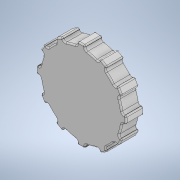
# Autodesk Inventor part: Dial_Radio
Saved by Autodesk Inventor 2021 (Build 250183000, 183)
## iProperties
Created: 2021-05-07
Part Number: Dial_Radio
Material: Generic
Document SubType Name: Modeling
Designer: trent
Density: 1 g/cm^3
Appearance: Default
Author: trent
Autodesk Inventor part; units mm, degrees
ref_plane "YZ Plane" through (0, 0, 0) normal (1, 0, 0) x (0, 1, 0)
ref_plane "XZ Plane" through (0, 0, 0) normal (0, 1, 0) x (-1, 0, 0)
ref_plane "XY Plane" through (0, 0, 0) normal (0, 0, 1) x (1, 0, 0)
sketch "Sketch1" plane through (0, 0, 0) normal (0, 0, 1) x (1, 0, 0)
  arc A0 (0.4789, 8.7369) -> (-0.5192, 8.7346) centre (0, 0) ccw
  line L0 (0.7133, 8.4304) -> (0.715, 8.4785)
  line L1 (-0.7524, 8.4247) -> (-0.7542, 8.4763)
  arc A1 (-0.5192, 8.7346) -> (-0.7542, 8.4763) centre (-0.5044, 8.485) ccw
  arc A2 (0.715, 8.4785) -> (0.4789, 8.7369) centre (0.4652, 8.4873) ccw
  arc A3 (-1.1785, 7.9127) -> (-0.7524, 8.4247) centre (-1.2521, 8.4073) ccw
  arc A4 (0.7133, 8.4304) -> (1.1417, 7.9181) centre (1.213, 8.413) ccw
  line L2 (-3.5975, 7.6577) -> (-3.62, 7.7001)
  line L3 (-4.864, 6.9198) -> (-4.8913, 6.9636)
  arc A5 (-4.8169, 7.3048) -> (-4.8913, 6.9636) centre (-4.6793, 7.0961) ccw
  arc A6 (-3.62, 7.7001) -> (-3.9537, 7.8058) centre (-3.8408, 7.5828) ccw
  arc A7 (-4.9769, 6.2634) -> (-4.864, 6.9198) centre (-5.288, 6.6549) ccw
  arc A8 (-3.9537, 7.8058) -> (-4.8169, 7.3048) centre (0, 0) ccw
  arc A9 (-3.5975, 7.6577) -> (-2.9703, 7.4281) centre (-3.156, 7.8924) ccw
  line L4 (-6.9443, 4.833) -> (-6.9851, 4.8585)
  line L5 (-7.6722, 3.5607) -> (-7.7178, 3.585)
  arc A10 (-7.824, 3.9176) -> (-7.7178, 3.585) centre (-7.6004, 3.8057) ccw
  arc A11 (-6.9851, 4.8585) -> (-7.3269, 4.7831) centre (-7.1176, 4.6465) ccw
  arc A12 (-7.4419, 2.9358) -> (-7.6722, 3.5607) centre (-7.907, 3.1193) ccw
  arc A13 (-7.3269, 4.7831) -> (-7.824, 3.9176) centre (0, 0) ccw
  arc A14 (-6.9443, 4.833) -> (-6.2864, 4.9478) centre (-6.6794, 5.257) ccw
  line L6 (-8.4304, 0.7133) -> (-8.4785, 0.715)
  line L7 (-8.4247, -0.7524) -> (-8.4763, -0.7542)
  arc A15 (-8.7346, -0.5192) -> (-8.4763, -0.7542) centre (-8.485, -0.5044) ccw
  arc A16 (-8.4785, 0.715) -> (-8.7369, 0.4789) centre (-8.4873, 0.4652) ccw
  arc A17 (-7.9127, -1.1785) -> (-8.4247, -0.7524) centre (-8.4073, -1.2521) ccw
  arc A18 (-8.7369, 0.4789) -> (-8.7346, -0.5192) centre (0, 0) ccw
  arc A19 (-8.4304, 0.7133) -> (-7.9181, 1.1417) centre (-8.413, 1.213) ccw
  line L8 (-7.6577, -3.5975) -> (-7.7001, -3.62)
  line L9 (-6.9198, -4.864) -> (-6.9636, -4.8913)
  arc A20 (-7.3048, -4.8169) -> (-6.9636, -4.8913) centre (-7.0961, -4.6793) ccw
  arc A21 (-7.7001, -3.62) -> (-7.8058, -3.9537) centre (-7.5828, -3.8408) ccw
  arc A22 (-6.2634, -4.9769) -> (-6.9198, -4.864) centre (-6.6549, -5.288) ccw
  arc A23 (-7.8058, -3.9537) -> (-7.3048, -4.8169) centre (0, 0) ccw
  arc A24 (-7.6577, -3.5975) -> (-7.4281, -2.9703) centre (-7.8924, -3.156) ccw
  line L10 (-4.833, -6.9443) -> (-4.8585, -6.9851)
  line L11 (-3.5607, -7.6722) -> (-3.585, -7.7178)
  arc A25 (-3.9176, -7.824) -> (-3.585, -7.7178) centre (-3.8057, -7.6004) ccw
  arc A26 (-4.8585, -6.9851) -> (-4.7831, -7.3269) centre (-4.6465, -7.1176) ccw
  arc A27 (-2.9358, -7.4419) -> (-3.5607, -7.6722) centre (-3.1193, -7.907) ccw
  arc A28 (-4.7831, -7.3269) -> (-3.9176, -7.824) centre (0, 0) ccw
  arc A29 (-4.833, -6.9443) -> (-4.9478, -6.2864) centre (-5.257, -6.6794) ccw
  line L12 (-0.7133, -8.4304) -> (-0.715, -8.4785)
  line L13 (0.7524, -8.4247) -> (0.7542, -8.4763)
  arc A30 (0.5192, -8.7346) -> (0.7542, -8.4763) centre (0.5044, -8.485) ccw
  arc A31 (-0.715, -8.4785) -> (-0.4789, -8.7369) centre (-0.4652, -8.4873) ccw
  arc A32 (1.1785, -7.9127) -> (0.7524, -8.4247) centre (1.2521, -8.4073) ccw
  arc A33 (-0.4789, -8.7369) -> (0.5192, -8.7346) centre (0, 0) ccw
  arc A34 (-0.7133, -8.4304) -> (-1.1417, -7.9181) centre (-1.213, -8.413) ccw
  line L14 (3.5975, -7.6577) -> (3.62, -7.7001)
  line L15 (4.864, -6.9198) -> (4.8913, -6.9636)
  arc A35 (4.8169, -7.3048) -> (4.8913, -6.9636) centre (4.6793, -7.0961) ccw
  arc A36 (3.62, -7.7001) -> (3.9537, -7.8058) centre (3.8408, -7.5828) ccw
  arc A37 (4.9769, -6.2634) -> (4.864, -6.9198) centre (5.288, -6.6549) ccw
  arc A38 (3.9537, -7.8058) -> (4.8169, -7.3048) centre (0, 0) ccw
  arc A39 (3.5975, -7.6577) -> (2.9703, -7.4281) centre (3.156, -7.8924) ccw
  line L16 (6.9443, -4.833) -> (6.9851, -4.8585)
  line L17 (7.6722, -3.5607) -> (7.7178, -3.585)
  arc A40 (7.824, -3.9176) -> (7.7178, -3.585) centre (7.6004, -3.8057) ccw
  arc A41 (6.9851, -4.8585) -> (7.3269, -4.7831) centre (7.1176, -4.6465) ccw
  arc A42 (7.4419, -2.9358) -> (7.6722, -3.5607) centre (7.907, -3.1193) ccw
  arc A43 (7.3269, -4.7831) -> (7.824, -3.9176) centre (0, 0) ccw
  arc A44 (6.9443, -4.833) -> (6.2864, -4.9478) centre (6.6794, -5.257) ccw
  line L18 (8.4304, -0.7133) -> (8.4785, -0.715)
  line L19 (8.4247, 0.7524) -> (8.4763, 0.7542)
  arc A45 (8.7346, 0.5192) -> (8.4763, 0.7542) centre (8.485, 0.5044) ccw
  arc A46 (8.4785, -0.715) -> (8.7369, -0.4789) centre (8.4873, -0.4652) ccw
  arc A47 (7.9127, 1.1785) -> (8.4247, 0.7524) centre (8.4073, 1.2521) ccw
  arc A48 (8.7369, -0.4789) -> (8.7346, 0.5192) centre (0, 0) ccw
  arc A49 (8.4304, -0.7133) -> (7.9181, -1.1417) centre (8.413, -1.213) ccw
  line L20 (7.6577, 3.5975) -> (7.7001, 3.62)
  line L21 (6.9198, 4.864) -> (6.9636, 4.8913)
  arc A50 (7.3048, 4.8169) -> (6.9636, 4.8913) centre (7.0961, 4.6793) ccw
  arc A51 (7.7001, 3.62) -> (7.8058, 3.9537) centre (7.5828, 3.8408) ccw
  arc A52 (6.2634, 4.9769) -> (6.9198, 4.864) centre (6.6549, 5.288) ccw
  arc A53 (7.8058, 3.9537) -> (7.3048, 4.8169) centre (0, 0) ccw
  arc A54 (7.6577, 3.5975) -> (7.4281, 2.9703) centre (7.8924, 3.156) ccw
  line L22 (4.833, 6.9443) -> (4.8585, 6.9851)
  line L23 (3.5607, 7.6722) -> (3.585, 7.7178)
  arc A55 (3.9176, 7.824) -> (3.585, 7.7178) centre (3.8057, 7.6004) ccw
  arc A56 (4.8585, 6.9851) -> (4.7831, 7.3269) centre (4.6465, 7.1176) ccw
  arc A57 (2.9358, 7.4419) -> (3.5607, 7.6722) centre (3.1193, 7.907) ccw
  arc A58 (4.7831, 7.3269) -> (3.9176, 7.824) centre (0, 0) ccw
  arc A59 (4.833, 6.9443) -> (4.9478, 6.2864) centre (5.257, 6.6794) ccw
  arc A60 (-1.1785, 7.9127) -> (-2.9703, 7.4281) centre (0, 0) ccw
  arc A61 (-4.9769, 6.2634) -> (-6.2864, 4.9478) centre (0, 0) ccw
  arc A62 (-7.4419, 2.9358) -> (-7.9181, 1.1417) centre (0, 0) ccw
  arc A63 (-7.9127, -1.1785) -> (-7.4281, -2.9703) centre (0, 0) ccw
  arc A64 (-6.2634, -4.9769) -> (-4.9478, -6.2864) centre (0, 0) ccw
  arc A65 (-2.9358, -7.4419) -> (-1.1417, -7.9181) centre (0, 0) ccw
  arc A66 (1.1785, -7.9127) -> (2.9703, -7.4281) centre (0, 0) ccw
  arc A67 (4.9769, -6.2634) -> (6.2864, -4.9478) centre (0, 0) ccw
  arc A68 (7.4419, -2.9358) -> (7.9181, -1.1417) centre (0, 0) ccw
  arc A69 (7.9127, 1.1785) -> (7.4281, 2.9703) centre (0, 0) ccw
  arc A70 (6.2634, 4.9769) -> (4.9478, 6.2864) centre (0, 0) ccw
  arc A71 (2.9358, 7.4419) -> (1.1417, 7.9181) centre (0, 0) ccw
  point P0 (0.7235, 8.72)
  point P1 (-0.7626, 8.7167)
  point P2 (0.6972, 7.9696)
  point P3 (-0.7364, 7.966)
  point P4 (-3.7335, 7.9135)
  point P5 (-5.0188, 7.1676)
  point P6 (-7.1901, 4.9865)
  point P7 (-7.9302, 3.6979)
  point P8 (-8.72, 0.7235)
  point P9 (-8.7167, -0.7626)
  point P10 (-7.9135, -3.7335)
  point P11 (-7.1676, -5.0188)
  point P12 (-4.9865, -7.1901)
  point P13 (-3.6979, -7.9302)
  point P14 (-0.7235, -8.72)
  point P15 (0.7626, -8.7167)
  point P16 (3.7335, -7.9135)
  point P17 (5.0188, -7.1676)
  point P18 (7.1901, -4.9865)
  point P19 (7.9302, -3.6979)
  point P20 (8.72, -0.7235)
  point P21 (8.7167, 0.7626)
  point P22 (7.9135, 3.7335)
  point P23 (7.1676, 5.0188)
  point P24 (4.9865, 7.1901)
  point P25 (3.6979, 7.9302)
  dimension "d1" = 17.5
  dimension "d4" = 0.25
  dimension "d5" = 0.5
  dimension "d8" = 360
  dimension "d10" = 8
  dimension "d11" = 4
  dimension "d12" = 0.8374
  dimension "d13" = 0.9159
  dimension "d14" = 8.4077
  dimension "d15" = 8.3542
  constraints: 168 point on circle, 72 centre point, 48 end point, 26 point on line, 8 tangent, 2 coincident, 2 equal radius, 265 other
  measures "d1" diameter of A0
  measures "d4" radius of A1
  measures "d5" radius of A3
  measures "d10" radius of A71
  measures "d11" angle of L18 L19
  measures "d12" distance between parallel lines of L18 L6
  measures "d13" distance between parallel lines of L7 L19
  measures "d14" distance from line of point (0.697, 7.97) L18
  measures "d15" distance from line of point (-0.736, 7.966) L18
extrude "Extrusion1" add sketch "Sketch1" along normal blind 3.5
fillet "Fillet1" radius 0.25 96 edges at (7.1493, 4.9236, 3.5) (6.9417, 4.8776, 3.5) (6.5701, 4.7952, 3.5) (5.6437, 5.67, 3.5) (4.7645, 6.5934, 3.5) (4.8457, 6.9647, 3.5) (4.8906, 7.1714, 3.5) (4.3575, 7.5878, 3.5) (3.7297, 7.8386, 3.5) (3.5729, 7.695, 3.5) (3.2922, 7.4378, 3.5) (2.0526, 7.7322, 3.5) (0.8294, 8.0923, 3.5) (0.7142, 8.4545, 3.5) (0.6497, 8.6559, 3.5) (-0.0202, 8.75, 3.5) (-0.6893, 8.6533, 3.5) (-0.7533, 8.4505, 3.5) (-0.8678, 8.0875, 3.5) (-2.0885, 7.7226, 3.5) (-3.3278, 7.4228, 3.5) (-3.6087, 7.6789, 3.5) (-3.7653, 7.8211, 3.5) (-4.3925, 7.5676, 3.5) (-4.9236, 7.1493, 3.5) (-4.8776, 6.9417, 3.5) (-4.7952, 6.5701, 3.5) (-5.67, 5.6437, 3.5) (-6.5934, 4.7645, 3.5) (-6.9647, 4.8457, 3.5) (-7.1714, 4.8906, 3.5) (-7.5878, 4.3575, 3.5) (-7.8386, 3.7297, 3.5) (-7.695, 3.5729, 3.5) (-7.4378, 3.2922, 3.5) (-7.7322, 2.0526, 3.5) (-8.0923, 0.8294, 3.5) (-8.4545, 0.7142, 3.5) (-8.6559, 0.6497, 3.5) (-8.75, -0.0202, 3.5) (-8.6533, -0.6893, 3.5) (-8.4505, -0.7533, 3.5) (-8.0875, -0.8678, 3.5) (-7.7226, -2.0885, 3.5) (-7.4228, -3.3278, 3.5) (-7.6789, -3.6087, 3.5) (-7.8211, -3.7653, 3.5) (-7.5676, -4.3925, 3.5) (-7.1493, -4.9236, 3.5) (-6.9417, -4.8776, 3.5) (-6.5701, -4.7952, 3.5) (-5.6437, -5.67, 3.5) (-4.7645, -6.5934, 3.5) (-4.8457, -6.9647, 3.5) (-4.8906, -7.1714, 3.5) (-4.3575, -7.5878, 3.5) (-3.7297, -7.8386, 3.5) (-3.5729, -7.695, 3.5) (-3.2922, -7.4378, 3.5) (-2.0526, -7.7322, 3.5) (-0.8294, -8.0923, 3.5) (-0.7142, -8.4545, 3.5) (-0.6497, -8.6559, 3.5) (0.0202, -8.75, 3.5) (0.6893, -8.6533, 3.5) (0.7533, -8.4505, 3.5) (0.8678, -8.0875, 3.5) (2.0885, -7.7226, 3.5) (3.3278, -7.4228, 3.5) (3.6087, -7.6789, 3.5) (3.7653, -7.8211, 3.5) (4.3925, -7.5676, 3.5) (4.9236, -7.1493, 3.5) (4.8776, -6.9417, 3.5) (4.7952, -6.5701, 3.5) (5.67, -5.6437, 3.5) (6.5934, -4.7645, 3.5) (6.9647, -4.8457, 3.5) (7.1714, -4.8906, 3.5) (7.5878, -4.3575, 3.5) (7.8386, -3.7297, 3.5) (7.695, -3.5729, 3.5) (7.4378, -3.2922, 3.5) (7.7322, -2.0526, 3.5) (8.0923, -0.8294, 3.5) (8.4545, -0.7142, 3.5) (8.6559, -0.6497, 3.5) (8.75, 0.0202, 3.5) (8.6533, 0.6893, 3.5) (8.4505, 0.7533, 3.5) (8.0875, 0.8678, 3.5) (7.7226, 2.0885, 3.5) (7.4228, 3.3278, 3.5) (7.6789, 3.6087, 3.5) (7.8211, 3.7653, 3.5) (7.5676, 4.3925, 3.5)
fillet "Fillet2" radius 0.25 96 edges at (7.1493, 4.9236, 0) (6.9417, 4.8776, 0) (6.5701, 4.7952, 0) (5.6437, 5.67, 0) (4.7645, 6.5934, 0) (4.8457, 6.9647, 0) (4.8906, 7.1714, 0) (4.3575, 7.5878, 0) (3.7297, 7.8386, 0) (3.5729, 7.695, 0) (3.2922, 7.4378, 0) (2.0526, 7.7322, 0) (0.8294, 8.0923, 0) (0.7142, 8.4545, 0) (0.6497, 8.6559, 0) (-0.0202, 8.75, 0) (-0.6893, 8.6533, 0) (-0.7533, 8.4505, 0) (-0.8678, 8.0875, 0) (-2.0885, 7.7226, 0) (-3.3278, 7.4228, 0) (-3.6087, 7.6789, 0) (-3.7653, 7.8211, 0) (-4.3925, 7.5676, 0) (-4.9236, 7.1493, 0) (-4.8776, 6.9417, 0) (-4.7952, 6.5701, 0) (-5.67, 5.6437, 0) (-6.5934, 4.7645, 0) (-6.9647, 4.8457, 0) (-7.1714, 4.8906, 0) (-7.5878, 4.3575, 0) (-7.8386, 3.7297, 0) (-7.695, 3.5729, 0) (-7.4378, 3.2922, 0) (-7.7322, 2.0526, 0) (-8.0923, 0.8294, 0) (-8.4545, 0.7142, 0) (-8.6559, 0.6497, 0) (-8.75, -0.0202, 0) (-8.6533, -0.6893, 0) (-8.4505, -0.7533, 0) (-8.0875, -0.8678, 0) (-7.7226, -2.0885, 0) (-7.4228, -3.3278, 0) (-7.6789, -3.6087, 0) (-7.8211, -3.7653, 0) (-7.5676, -4.3925, 0) (-7.1493, -4.9236, 0) (-6.9417, -4.8776, 0) (-6.5701, -4.7952, 0) (-5.6437, -5.67, 0) (-4.7645, -6.5934, 0) (-4.8457, -6.9647, 0) (-4.8906, -7.1714, 0) (-4.3575, -7.5878, 0) (-3.7297, -7.8386, 0) (-3.5729, -7.695, 0) (-3.2922, -7.4378, 0) (-2.0526, -7.7322, 0) (-0.8294, -8.0923, 0) (-0.7142, -8.4545, 0) (-0.6497, -8.6559, 0) (0.0202, -8.75, 0) (0.6893, -8.6533, 0) (0.7533, -8.4505, 0) (0.8678, -8.0875, 0) (2.0885, -7.7226, 0) (3.3278, -7.4228, 0) (3.6087, -7.6789, 0) (3.7653, -7.8211, 0) (4.3925, -7.5676, 0) (4.9236, -7.1493, 0) (4.8776, -6.9417, 0) (4.7952, -6.5701, 0) (5.67, -5.6437, 0) (6.5934, -4.7645, 0) (6.9647, -4.8457, 0) (7.1714, -4.8906, 0) (7.5878, -4.3575, 0) (7.8386, -3.7297, 0) (7.695, -3.5729, 0) (7.4378, -3.2922, 0) (7.7322, -2.0526, 0) (8.0923, -0.8294, 0) (8.4545, -0.7142, 0) (8.6559, -0.6497, 0) (8.75, 0.0202, 0) (8.6533, 0.6893, 0) (8.4505, 0.7533, 0) (8.0875, 0.8678, 0) (7.7226, 2.0885, 0) (7.4228, 3.3278, 0) (7.6789, 3.6087, 0) (7.8211, 3.7653, 0) (7.5676, 4.3925, 0)
body "Solid1"
